Autodesk Inventor part; units mm, degrees
(part 2 of 3)
sketch "Sketch1" plane through (0, 0, 0) normal (0, 1, 0) x (-1, 0, 0)
  line L0 (1.875, 1.875) -> (-1.875, -1.875) construction
  circle A0 centre (0, 0) radius 5 projected
  circle A1 centre (0, 0) radius 7.7717
  line L1 (3.8714, 3.1643) -> (5.8376, 5.1305)
  line L2 (3.1643, 3.8714) -> (5.1305, 5.8376)
  line L3 (-3.1643, -3.8714) -> (-5.1305, -5.8376)
  line L4 (-3.8714, -3.1643) -> (-5.8376, -5.1305)
  line L5 (3.1643, -3.8714) -> (5.1305, -5.8376)
  line L6 (5.8376, -5.1305) -> (3.8714, -3.1643)
  line L7 (-3.8714, 3.1643) -> (-5.8376, 5.1305)
  line L8 (-3.1643, 3.8714) -> (-5.1305, 5.8376)
  line L9 (8.418, 2.4779) -> (8.489, 2.3785)
  line L10 (8.489, 2.3785) -> (8.5402, 2.3467)
  line L11 (8.5402, 2.3467) -> (8.588, 2.3267)
  line L12 (8.588, 2.3267) -> (8.6339, 2.3133)
  line L13 (8.6339, 2.3133) -> (8.6785, 2.3043)
  line L14 (8.6785, 2.3043) -> (8.7654, 2.2952)
  line L15 (8.7654, 2.2952) -> (8.8499, 2.2948)
  line L16 (8.8499, 2.2948) -> (8.9327, 2.3008)
  line L17 (8.9327, 2.3008) -> (9.0141, 2.3121)
  line L18 (9.0141, 2.3121) -> (9.1751, 2.3417)
  line L19 (9.1751, 2.3417) -> (9.3406, 2.3535)
  line L20 (9.3406, 2.3535) -> (9.5094, 2.3516)
  line L21 (9.5094, 2.3516) -> (9.6806, 2.3391)
  line L22 (9.6806, 2.3391) -> (9.8537, 2.3172)
  line L23 (9.8537, 2.3172) -> (10.0284, 2.2867)
  line L24 (10.0284, 2.2867) -> (10.2044, 2.2482)
  line L25 (10.2044, 2.2482) -> (10.3815, 2.202)
  line L26 (10.3815, 2.202) -> (10.5594, 2.1484)
  line L27 (10.5594, 2.1484) -> (10.7381, 2.0875)
  line L28 (10.7381, 2.0875) -> (10.9172, 2.0196)
  line L29 (10.9172, 2.0196) -> (11.0517, 1.9642)
  line L30 (11.0517, 1.9642) -> (11.1178, 1.5471)
  line L31 (11.1178, 1.5471) -> (11.007, 1.4528)
  line L32 (11.007, 1.4528) -> (10.8576, 1.3329)
  line L33 (10.8576, 1.3329) -> (10.7065, 1.2198)
  line L34 (10.7065, 1.2198) -> (10.5538, 1.1138)
  line L35 (10.5538, 1.1138) -> (10.3997, 1.0152)
  line L36 (10.3997, 1.0152) -> (10.2442, 0.9241)
  line L37 (10.2442, 0.9241) -> (10.0875, 0.8412)
  line L38 (10.0875, 0.8412) -> (9.9296, 0.7669)
  line L39 (9.9296, 0.7669) -> (9.7707, 0.702)
  line L40 (9.7707, 0.702) -> (9.6107, 0.6481)
  line L41 (9.6107, 0.6481) -> (9.4497, 0.6082)
  line L42 (9.4497, 0.6082) -> (9.2874, 0.5866)
  line L43 (9.2874, 0.5866) -> (9.2065, 0.5721)
  line L44 (9.2065, 0.5721) -> (9.1259, 0.5523)
  line L45 (9.1259, 0.5523) -> (9.0456, 0.5258)
  line L46 (9.0456, 0.5258) -> (8.9658, 0.4903)
  line L47 (8.9658, 0.4903) -> (8.9262, 0.4679)
  line L48 (8.9262, 0.4679) -> (8.8867, 0.441)
  line L49 (8.8867, 0.441) -> (8.8474, 0.4073)
  line L50 (8.8474, 0.4073) -> (8.8085, 0.3612)
  line L51 (8.8085, 0.3612) -> (8.7717, 0.2447)
  line L52 (8.7717, 0.2447) -> (8.7717, -0.2447)
  line L53 (8.7717, -0.2447) -> (8.8085, -0.3612)
  line L54 (8.8085, -0.3612) -> (8.8474, -0.4073)
  line L55 (8.8474, -0.4073) -> (8.8867, -0.441)
  line L56 (8.8867, -0.441) -> (8.9262, -0.4679)
  line L57 (8.9262, -0.4679) -> (8.9658, -0.4903)
  line L58 (8.9658, -0.4903) -> (9.0456, -0.5258)
  line L59 (9.0456, -0.5258) -> (9.1259, -0.5523)
  line L60 (9.1259, -0.5523) -> (9.2065, -0.5721)
  line L61 (9.2065, -0.5721) -> (9.2874, -0.5866)
  line L62 (9.2874, -0.5866) -> (9.4497, -0.6082)
  line L63 (9.4497, -0.6082) -> (9.6107, -0.6481)
  line L64 (9.6107, -0.6481) -> (9.7707, -0.702)
  line L65 (9.7707, -0.702) -> (9.9296, -0.7669)
  line L66 (9.9296, -0.7669) -> (10.0875, -0.8412)
  line L67 (10.0875, -0.8412) -> (10.2442, -0.9241)
  line L68 (10.2442, -0.9241) -> (10.3997, -1.0152)
  line L69 (10.3997, -1.0152) -> (10.5538, -1.1138)
  line L70 (10.5538, -1.1138) -> (10.7065, -1.2198)
  line L71 (10.7065, -1.2198) -> (10.8576, -1.3329)
  line L72 (10.8576, -1.3329) -> (11.007, -1.4528)
  line L73 (11.007, -1.4528) -> (11.1178, -1.5471)
  line L74 (11.1178, -1.5471) -> (11.0517, -1.9642)
  line L75 (11.0517, -1.9642) -> (10.9172, -2.0197)
  line L76 (10.9172, -2.0197) -> (10.7381, -2.0875)
  line L77 (10.7381, -2.0875) -> (10.5594, -2.1484)
  line L78 (10.5594, -2.1484) -> (10.3815, -2.202)
  line L79 (10.3815, -2.202) -> (10.2044, -2.2482)
  line L80 (10.2044, -2.2482) -> (10.0284, -2.2867)
  line L81 (10.0284, -2.2867) -> (9.8537, -2.3172)
  line L82 (9.8537, -2.3172) -> (9.6806, -2.3391)
  line L83 (9.6806, -2.3391) -> (9.5094, -2.3516)
  line L84 (9.5094, -2.3516) -> (9.3406, -2.3535)
  line L85 (9.3406, -2.3535) -> (9.1751, -2.3417)
  line L86 (9.1751, -2.3417) -> (9.0141, -2.3121)
  line L87 (9.0141, -2.3121) -> (8.9327, -2.3008)
  line L88 (8.9327, -2.3008) -> (8.8499, -2.2948)
  line L89 (8.8499, -2.2948) -> (8.7654, -2.2952)
  line L90 (8.7654, -2.2952) -> (8.6786, -2.3043)
  line L91 (8.6786, -2.3043) -> (8.6339, -2.3133)
  line L92 (8.6339, -2.3133) -> (8.588, -2.3268)
  line L93 (8.588, -2.3268) -> (8.5402, -2.3467)
  line L94 (8.5402, -2.3467) -> (8.489, -2.3785)
  line L95 (8.489, -2.3785) -> (8.418, -2.4779)
  line L96 (8.418, -2.4779) -> (8.2667, -2.9433)
  line L97 (8.2667, -2.9433) -> (8.2658, -3.0655)
  line L98 (8.2658, -3.0655) -> (8.2885, -3.1213)
  line L99 (8.2885, -3.1213) -> (8.3154, -3.1655)
  line L100 (8.3154, -3.1655) -> (8.3447, -3.2034)
  line L101 (8.3447, -3.2034) -> (8.3755, -3.2369)
  line L102 (8.3755, -3.2369) -> (8.4404, -3.2953)
  line L103 (8.4404, -3.2953) -> (8.5086, -3.3453)
  line L104 (8.5086, -3.3453) -> (8.5791, -3.3891)
  line L105 (8.5791, -3.3891) -> (8.6515, -3.4279)
  line L106 (8.6515, -3.4279) -> (8.7992, -3.4985)
  line L107 (8.7992, -3.4985) -> (8.94, -3.5863)
  line L108 (8.94, -3.5863) -> (9.0755, -3.687)
  line L109 (9.0755, -3.687) -> (9.2066, -3.7977)
  line L110 (9.2066, -3.7977) -> (9.3338, -3.9172)
  line L111 (9.3338, -3.9172) -> (9.4573, -4.0445)
  line L112 (9.4573, -4.0445) -> (9.577, -4.1792)
  line L113 (9.577, -4.1792) -> (9.6931, -4.3206)
  line L114 (9.6931, -4.3206) -> (9.8055, -4.4686)
  line L115 (9.8055, -4.4686) -> (9.9143, -4.6228)
  line L116 (9.9143, -4.6228) -> (10.0193, -4.783)
  line L117 (10.0193, -4.783) -> (10.0956, -4.907)
  line L118 (10.0956, -4.907) -> (9.9038, -5.2832)
  line L119 (9.9038, -5.2832) -> (9.7587, -5.2944)
  line L120 (9.7587, -5.2944) -> (9.5674, -5.3036)
  line L121 (9.5674, -5.3036) -> (9.3788, -5.3063)
  line L122 (9.3788, -5.3063) -> (9.1929, -5.3023)
  line L123 (9.1929, -5.3023) -> (9.0102, -5.2915)
  line L124 (9.0102, -5.2915) -> (8.8309, -5.2738)
  line L125 (8.8309, -5.2738) -> (8.6554, -5.2487)
  line L126 (8.6554, -5.2487) -> (8.484, -5.2161)
  line L127 (8.484, -5.2161) -> (8.3173, -5.1751)
  line L128 (8.3173, -5.1751) -> (8.1562, -5.1247)
  line L129 (8.1562, -5.1247) -> (8.0024, -5.0624)
  line L130 (8.0024, -5.0624) -> (7.8585, -4.9844)
  line L131 (7.8585, -4.9844) -> (7.7845, -4.9486)
  line L132 (7.7845, -4.9486) -> (7.7076, -4.9173)
  line L133 (7.7076, -4.9173) -> (7.6271, -4.8915)
  line L134 (7.6271, -4.8915) -> (7.5417, -4.8733)
  line L135 (7.5417, -4.8733) -> (7.4964, -4.8681)
  line L136 (7.4964, -4.8681) -> (7.4486, -4.8667)
  line L137 (7.4486, -4.8667) -> (7.3971, -4.8709)
  line L138 (7.3971, -4.8709) -> (7.3385, -4.8853)
  line L139 (7.3385, -4.8853) -> (7.2403, -4.9579)
  line L140 (7.2403, -4.9579) -> (6.9526, -5.3538)
  line L141 (6.9526, -5.3538) -> (6.914, -5.4697)
  line L142 (6.914, -5.4697) -> (6.9183, -5.5298)
  line L143 (6.9183, -5.5298) -> (6.9303, -5.5802)
  line L144 (6.9303, -5.5802) -> (6.9464, -5.6252)
  line L145 (6.9464, -5.6252) -> (6.9653, -5.6667)
  line L146 (6.9653, -5.6667) -> (7.009, -5.7423)
  line L147 (7.009, -5.7423) -> (7.0584, -5.8109)
  line L148 (7.0584, -5.8109) -> (7.1119, -5.8743)
  line L149 (7.1119, -5.8743) -> (7.1688, -5.9336)
  line L150 (7.1688, -5.9336) -> (7.2875, -6.0464)
  line L151 (7.2875, -6.0464) -> (7.3943, -6.1734)
  line L152 (7.3943, -6.1734) -> (7.492, -6.311)
  line L153 (7.492, -6.311) -> (7.5825, -6.4569)
  line L154 (7.5825, -6.4569) -> (7.6665, -6.6098)
  line L155 (7.6665, -6.6098) -> (7.7445, -6.769)
  line L156 (7.7445, -6.769) -> (7.8168, -6.9341)
  line L157 (7.8168, -6.9341) -> (7.8835, -7.1045)
  line L158 (7.8835, -7.1045) -> (7.9447, -7.28)
  line L159 (7.9447, -7.28) -> (8.0005, -7.4603)
  line L160 (8.0005, -7.4603) -> (8.0509, -7.6451)
  line L161 (8.0509, -7.6451) -> (8.0851, -7.7865)
  line L162 (8.0851, -7.7865) -> (7.7865, -8.0851)
  line L163 (7.7865, -8.0851) -> (7.6451, -8.0509)
  line L164 (7.6451, -8.0509) -> (7.4603, -8.0005)
  line L165 (7.4603, -8.0005) -> (7.28, -7.9447)
  line L166 (7.28, -7.9447) -> (7.1045, -7.8835)
  line L167 (7.1045, -7.8835) -> (6.9341, -7.8168)
  line L168 (6.9341, -7.8168) -> (6.769, -7.7445)
  line L169 (6.769, -7.7445) -> (6.6098, -7.6665)
  line L170 (6.6098, -7.6665) -> (6.4569, -7.5825)
  line L171 (6.4569, -7.5825) -> (6.311, -7.492)
  line L172 (6.311, -7.492) -> (6.1734, -7.3943)
  line L173 (6.1734, -7.3943) -> (6.0464, -7.2875)
  line L174 (6.0464, -7.2875) -> (5.9336, -7.1688)
  line L175 (5.9336, -7.1688) -> (5.8743, -7.1119)
  line L176 (5.8743, -7.1119) -> (5.8109, -7.0584)
  line L177 (5.8109, -7.0584) -> (5.7423, -7.009)
  line L178 (5.7423, -7.009) -> (5.6667, -6.9653)
  line L179 (5.6667, -6.9653) -> (5.6252, -6.9464)
  line L180 (5.6252, -6.9464) -> (5.5802, -6.9303)
  line L181 (5.5802, -6.9303) -> (5.5298, -6.9183)
  line L182 (5.5298, -6.9183) -> (5.4697, -6.9139)
  line L183 (5.4697, -6.9139) -> (5.3538, -6.9526)
  line L184 (5.3538, -6.9526) -> (4.9579, -7.2403)
  line L185 (4.9579, -7.2403) -> (4.8853, -7.3385)
  line L186 (4.8853, -7.3385) -> (4.8709, -7.3971)
  line L187 (4.8709, -7.3971) -> (4.8667, -7.4486)
  line L188 (4.8667, -7.4486) -> (4.8681, -7.4965)
  line L189 (4.8681, -7.4965) -> (4.8733, -7.5417)
  line L190 (4.8733, -7.5417) -> (4.8915, -7.6271)
  line L191 (4.8915, -7.6271) -> (4.9172, -7.7076)
  line L192 (4.9172, -7.7076) -> (4.9486, -7.7845)
  line L193 (4.9486, -7.7845) -> (4.9844, -7.8585)
  line L194 (4.9844, -7.8585) -> (5.0624, -8.0024)
  line L195 (5.0624, -8.0024) -> (5.1247, -8.1562)
  line L196 (5.1247, -8.1562) -> (5.1751, -8.3173)
  line L197 (5.1751, -8.3173) -> (5.2161, -8.484)
  line L198 (5.2161, -8.484) -> (5.2487, -8.6554)
  line L199 (5.2487, -8.6554) -> (5.2738, -8.8309)
  line L200 (5.2738, -8.8309) -> (5.2915, -9.0102)
  line L201 (5.2915, -9.0102) -> (5.3023, -9.1929)
  line L202 (5.3023, -9.1929) -> (5.3063, -9.3788)
  line L203 (5.3063, -9.3788) -> (5.3036, -9.5674)
  line L204 (5.3036, -9.5674) -> (5.2944, -9.7587)
  line L205 (5.2944, -9.7587) -> (5.2832, -9.9038)
  line L206 (5.2832, -9.9038) -> (4.907, -10.0956)
  line L207 (4.907, -10.0956) -> (4.783, -10.0193)
  line L208 (4.783, -10.0193) -> (4.6228, -9.9143)
  line L209 (4.6228, -9.9143) -> (4.4686, -9.8055)
  line L210 (4.4686, -9.8055) -> (4.3207, -9.6931)
  line L211 (4.3207, -9.6931) -> (4.1792, -9.577)
  line L212 (4.1792, -9.577) -> (4.0445, -9.4572)
  line L213 (4.0445, -9.4572) -> (3.9172, -9.3338)
  line L214 (3.9172, -9.3338) -> (3.7977, -9.2066)
  line L215 (3.7977, -9.2066) -> (3.687, -9.0755)
  line L216 (3.687, -9.0755) -> (3.5863, -8.94)
  line L217 (3.5863, -8.94) -> (3.4985, -8.7992)
  line L218 (3.4985, -8.7992) -> (3.4279, -8.6515)
  line L219 (3.4279, -8.6515) -> (3.3891, -8.5791)
  line L220 (3.3891, -8.5791) -> (3.3453, -8.5086)
  line L221 (3.3453, -8.5086) -> (3.2953, -8.4404)
  line L222 (3.2953, -8.4404) -> (3.2369, -8.3755)
  line L223 (3.2369, -8.3755) -> (3.2033, -8.3447)
  line L224 (3.2033, -8.3447) -> (3.1655, -8.3154)
  line L225 (3.1655, -8.3154) -> (3.1213, -8.2885)
  line L226 (3.1213, -8.2885) -> (3.0655, -8.2658)
  line L227 (3.0655, -8.2658) -> (2.9433, -8.2667)
  line L228 (2.9433, -8.2667) -> (2.4779, -8.418)
  line L229 (2.4779, -8.418) -> (2.3785, -8.489)
  line L230 (2.3785, -8.489) -> (2.3467, -8.5402)
  line L231 (2.3467, -8.5402) -> (2.3267, -8.588)
  line L232 (2.3267, -8.588) -> (2.3133, -8.6339)
  line L233 (2.3133, -8.6339) -> (2.3043, -8.6785)
  line L234 (2.3043, -8.6785) -> (2.2952, -8.7654)
  line L235 (2.2952, -8.7654) -> (2.2948, -8.8499)
  line L236 (2.2948, -8.8499) -> (2.3008, -8.9327)
  line L237 (2.3008, -8.9327) -> (2.3121, -9.0141)
  line L238 (2.3121, -9.0141) -> (2.3417, -9.1751)
  line L239 (2.3417, -9.1751) -> (2.3535, -9.3406)
  line L240 (2.3535, -9.3406) -> (2.3516, -9.5094)
  line L241 (2.3516, -9.5094) -> (2.3391, -9.6806)
  line L242 (2.3391, -9.6806) -> (2.3172, -9.8537)
  line L243 (2.3172, -9.8537) -> (2.2867, -10.0284)
  line L244 (2.2867, -10.0284) -> (2.2482, -10.2044)
  line L245 (2.2482, -10.2044) -> (2.202, -10.3815)
  line L246 (2.202, -10.3815) -> (2.1484, -10.5594)
  line L247 (2.1484, -10.5594) -> (2.0875, -10.7381)
  line L248 (2.0875, -10.7381) -> (2.0196, -10.9172)
  line L249 (2.0196, -10.9172) -> (1.9642, -11.0517)
  line L250 (1.9642, -11.0517) -> (1.5471, -11.1178)
  line L251 (1.5471, -11.1178) -> (1.4528, -11.007)
  line L252 (1.4528, -11.007) -> (1.3329, -10.8576)
  line L253 (1.3329, -10.8576) -> (1.2198, -10.7065)
  line L254 (1.2198, -10.7065) -> (1.1138, -10.5538)
  line L255 (1.1138, -10.5538) -> (1.0152, -10.3997)
  line L256 (1.0152, -10.3997) -> (0.9241, -10.2442)
  line L257 (0.9241, -10.2442) -> (0.8412, -10.0875)
  line L258 (0.8412, -10.0875) -> (0.7669, -9.9296)
  line L259 (0.7669, -9.9296) -> (0.702, -9.7707)
  line L260 (0.702, -9.7707) -> (0.6481, -9.6107)
  line L261 (0.6481, -9.6107) -> (0.6082, -9.4497)
  line L262 (0.6082, -9.4497) -> (0.5866, -9.2874)
  line L263 (0.5866, -9.2874) -> (0.5721, -9.2065)
  line L264 (0.5721, -9.2065) -> (0.5523, -9.1259)
  line L265 (0.5523, -9.1259) -> (0.5258, -9.0456)
  line L266 (0.5258, -9.0456) -> (0.4903, -8.9658)
  line L267 (0.4903, -8.9658) -> (0.4679, -8.9262)
  line L268 (0.4679, -8.9262) -> (0.441, -8.8867)
  line L269 (0.441, -8.8867) -> (0.4073, -8.8474)
  line L270 (0.4073, -8.8474) -> (0.3612, -8.8085)
  line L271 (0.3612, -8.8085) -> (0.2447, -8.7717)
  line L272 (0.2447, -8.7717) -> (-0.2447, -8.7717)
  line L273 (-0.2447, -8.7717) -> (-0.3612, -8.8085)
  line L274 (-0.3612, -8.8085) -> (-0.4073, -8.8474)
  line L275 (-0.4073, -8.8474) -> (-0.441, -8.8866)
  line L276 (-0.441, -8.8866) -> (-0.4679, -8.9262)
  line L277 (-0.4679, -8.9262) -> (-0.4903, -8.9658)
  line L278 (-0.4903, -8.9658) -> (-0.5258, -9.0456)
  line L279 (-0.5258, -9.0456) -> (-0.5523, -9.1259)
  line L280 (-0.5523, -9.1259) -> (-0.5721, -9.2065)
  line L281 (-0.5721, -9.2065) -> (-0.5866, -9.2874)
  line L282 (-0.5866, -9.2874) -> (-0.6082, -9.4497)
  line L283 (-0.6082, -9.4497) -> (-0.6481, -9.6107)
  line L284 (-0.6481, -9.6107) -> (-0.702, -9.7707)
  line L285 (-0.702, -9.7707) -> (-0.7669, -9.9296)
  line L286 (-0.7669, -9.9296) -> (-0.8412, -10.0875)
  line L287 (-0.8412, -10.0875) -> (-0.9241, -10.2442)
  line L288 (-0.9241, -10.2442) -> (-1.0152, -10.3997)
  line L289 (-1.0152, -10.3997) -> (-1.1138, -10.5538)
  line L290 (-1.1138, -10.5538) -> (-1.2198, -10.7065)
  line L291 (-1.2198, -10.7065) -> (-1.3329, -10.8576)
  line L292 (-1.3329, -10.8576) -> (-1.4528, -11.007)
  line L293 (-1.4528, -11.007) -> (-1.5471, -11.1178)
  line L294 (-1.5471, -11.1178) -> (-1.9642, -11.0517)
  line L295 (-1.9642, -11.0517) -> (-2.0197, -10.9172)
  line L296 (-2.0197, -10.9172) -> (-2.0875, -10.7381)
  line L297 (-2.0875, -10.7381) -> (-2.1484, -10.5594)
  line L298 (-2.1484, -10.5594) -> (-2.202, -10.3815)
  line L299 (-2.202, -10.3815) -> (-2.2482, -10.2044)
  line L300 (-2.2482, -10.2044) -> (-2.2867, -10.0284)
  line L301 (-2.2867, -10.0284) -> (-2.3172, -9.8537)
  line L302 (-2.3172, -9.8537) -> (-2.3391, -9.6806)
  line L303 (-2.3391, -9.6806) -> (-2.3516, -9.5094)
  line L304 (-2.3516, -9.5094) -> (-2.3535, -9.3406)
  line L305 (-2.3535, -9.3406) -> (-2.3417, -9.1751)
  line L306 (-2.3417, -9.1751) -> (-2.3121, -9.0141)
  line L307 (-2.3121, -9.0141) -> (-2.3008, -8.9327)
  line L308 (-2.3008, -8.9327) -> (-2.2948, -8.8499)
  line L309 (-2.2948, -8.8499) -> (-2.2952, -8.7654)
  line L310 (-2.2952, -8.7654) -> (-2.3043, -8.6785)
  line L311 (-2.3043, -8.6785) -> (-2.3133, -8.6339)
  line L312 (-2.3133, -8.6339) -> (-2.3267, -8.588)
  line L313 (-2.3267, -8.588) -> (-2.3467, -8.5402)
  line L314 (-2.3467, -8.5402) -> (-2.3785, -8.489)
  line L315 (-2.3785, -8.489) -> (-2.4779, -8.418)
  line L316 (-2.4779, -8.418) -> (-2.9433, -8.2667)
  line L317 (-2.9433, -8.2667) -> (-3.0655, -8.2658)
  line L318 (-3.0655, -8.2658) -> (-3.1213, -8.2885)
  line L319 (-3.1213, -8.2885) -> (-3.1655, -8.3154)
  line L320 (-3.1655, -8.3154) -> (-3.2033, -8.3447)
  line L321 (-3.2033, -8.3447) -> (-3.2369, -8.3755)
  line L322 (-3.2369, -8.3755) -> (-3.2953, -8.4404)
  line L323 (-3.2953, -8.4404) -> (-3.3453, -8.5086)
  line L324 (-3.3453, -8.5086) -> (-3.3891, -8.5791)
  line L325 (-3.3891, -8.5791) -> (-3.4279, -8.6515)
  line L326 (-3.4279, -8.6515) -> (-3.4985, -8.7992)
  line L327 (-3.4985, -8.7992) -> (-3.5863, -8.94)
  line L328 (-3.5863, -8.94) -> (-3.687, -9.0755)
  line L329 (-3.687, -9.0755) -> (-3.7977, -9.2066)
  line L330 (-3.7977, -9.2066) -> (-3.9172, -9.3338)
  line L331 (-3.9172, -9.3338) -> (-4.0445, -9.4572)
  line L332 (-4.0445, -9.4572) -> (-4.1792, -9.577)
  line L333 (-4.1792, -9.577) -> (-4.3206, -9.6931)
  line L334 (-4.3206, -9.6931) -> (-4.4686, -9.8055)
  line L335 (-4.4686, -9.8055) -> (-4.6228, -9.9143)
  line L336 (-4.6228, -9.9143) -> (-4.783, -10.0193)
  line L337 (-4.783, -10.0193) -> (-4.907, -10.0956)
  line L338 (-4.907, -10.0956) -> (-5.2832, -9.9038)
  line L339 (-5.2832, -9.9038) -> (-5.2944, -9.7587)
  line L340 (-5.2944, -9.7587) -> (-5.3036, -9.5674)
  line L341 (-5.3036, -9.5674) -> (-5.3063, -9.3788)
  line L342 (-5.3063, -9.3788) -> (-5.3023, -9.1929)
  line L343 (-5.3023, -9.1929) -> (-5.2915, -9.0102)
  line L344 (-5.2915, -9.0102) -> (-5.2738, -8.8309)
  line L345 (-5.2738, -8.8309) -> (-5.2487, -8.6554)
  line L346 (-5.2487, -8.6554) -> (-5.2161, -8.484)
  line L347 (-5.2161, -8.484) -> (-5.1751, -8.3173)
  line L348 (-5.1751, -8.3173) -> (-5.1247, -8.1562)
  line L349 (-5.1247, -8.1562) -> (-5.0624, -8.0024)
  line L350 (-5.0624, -8.0024) -> (-4.9844, -7.8584)
  line L351 (-4.9844, -7.8584) -> (-4.9486, -7.7845)
  line L352 (-4.9486, -7.7845) -> (-4.9173, -7.7076)
  line L353 (-4.9173, -7.7076) -> (-4.8915, -7.6271)
  line L354 (-4.8915, -7.6271) -> (-4.8733, -7.5417)
  line L355 (-4.8733, -7.5417) -> (-4.8681, -7.4965)
  line L356 (-4.8681, -7.4965) -> (-4.8667, -7.4486)
  line L357 (-4.8667, -7.4486) -> (-4.8709, -7.3971)
  line L358 (-4.8709, -7.3971) -> (-4.8853, -7.3385)
  line L359 (-4.8853, -7.3385) -> (-4.9579, -7.2403)
  line L360 (-4.9579, -7.2403) -> (-5.3538, -6.9526)
  line L361 (-5.3538, -6.9526) -> (-5.4697, -6.914)
  line L362 (-5.4697, -6.914) -> (-5.5298, -6.9183)
  line L363 (-5.5298, -6.9183) -> (-5.5802, -6.9303)
  line L364 (-5.5802, -6.9303) -> (-5.6252, -6.9464)
  line L365 (-5.6252, -6.9464) -> (-5.6667, -6.9653)
  line L366 (-5.6667, -6.9653) -> (-5.7423, -7.009)
  line L367 (-5.7423, -7.009) -> (-5.8109, -7.0584)
  line L368 (-5.8109, -7.0584) -> (-5.8743, -7.1119)
  line L369 (-5.8743, -7.1119) -> (-5.9336, -7.1688)
  line L370 (-5.9336, -7.1688) -> (-6.0464, -7.2875)
  line L371 (-6.0464, -7.2875) -> (-6.1734, -7.3943)
  line L372 (-6.1734, -7.3943) -> (-6.311, -7.492)
  line L373 (-6.311, -7.492) -> (-6.4569, -7.5825)
  line L374 (-6.4569, -7.5825) -> (-6.6098, -7.6665)
  line L375 (-6.6098, -7.6665) -> (-6.769, -7.7445)
  line L376 (-6.769, -7.7445) -> (-6.9341, -7.8168)
  line L377 (-6.9341, -7.8168) -> (-7.1045, -7.8835)
  line L378 (-7.1045, -7.8835) -> (-7.28, -7.9447)
  line L379 (-7.28, -7.9447) -> (-7.4603, -8.0005)
  line L380 (-7.4603, -8.0005) -> (-7.6451, -8.0509)
  line L381 (-7.6451, -8.0509) -> (-7.7865, -8.0851)
  line L382 (-7.7865, -8.0851) -> (-8.0851, -7.7865)
  line L383 (-8.0851, -7.7865) -> (-8.0509, -7.6451)
  line L384 (-8.0509, -7.6451) -> (-8.0005, -7.4603)
  line L385 (-8.0005, -7.4603) -> (-7.9447, -7.28)
  line L386 (-7.9447, -7.28) -> (-7.8835, -7.1045)
  line L387 (-7.8835, -7.1045) -> (-7.8168, -6.9341)
  line L388 (-7.8168, -6.9341) -> (-7.7445, -6.769)
  line L389 (-7.7445, -6.769) -> (-7.6665, -6.6098)
  line L390 (-7.6665, -6.6098) -> (-7.5825, -6.4569)
  line L391 (-7.5825, -6.4569) -> (-7.492, -6.311)
  line L392 (-7.492, -6.311) -> (-7.3943, -6.1734)
  line L393 (-7.3943, -6.1734) -> (-7.2875, -6.0464)
  line L394 (-7.2875, -6.0464) -> (-7.1688, -5.9336)
  line L395 (-7.1688, -5.9336) -> (-7.1119, -5.8743)
  line L396 (-7.1119, -5.8743) -> (-7.0584, -5.8108)
  line L397 (-7.0584, -5.8108) -> (-7.009, -5.7423)
  line L398 (-7.009, -5.7423) -> (-6.9653, -5.6667)
  line L399 (-6.9653, -5.6667) -> (-6.9464, -5.6252)
  line L400 (-6.9464, -5.6252) -> (-6.9303, -5.5802)
  line L401 (-6.9303, -5.5802) -> (-6.9183, -5.5298)
  line L402 (-6.9183, -5.5298) -> (-6.9139, -5.4697)
  line L403 (-6.9139, -5.4697) -> (-6.9526, -5.3538)
  line L404 (-6.9526, -5.3538) -> (-7.2403, -4.9579)
  line L405 (-7.2403, -4.9579) -> (-7.3385, -4.8853)
  line L406 (-7.3385, -4.8853) -> (-7.3971, -4.8709)
  line L407 (-7.3971, -4.8709) -> (-7.4486, -4.8667)
  line L408 (-7.4486, -4.8667) -> (-7.4965, -4.8681)
  line L409 (-7.4965, -4.8681) -> (-7.5417, -4.8733)
  line L410 (-7.5417, -4.8733) -> (-7.6271, -4.8915)
  line L411 (-7.6271, -4.8915) -> (-7.7076, -4.9173)
  line L412 (-7.7076, -4.9173) -> (-7.7845, -4.9486)
  line L413 (-7.7845, -4.9486) -> (-7.8585, -4.9844)
  line L414 (-7.8585, -4.9844) -> (-8.0024, -5.0624)
  line L415 (-8.0024, -5.0624) -> (-8.1562, -5.1247)
  line L416 (-8.1562, -5.1247) -> (-8.3173, -5.1751)
  line L417 (-8.3173, -5.1751) -> (-8.484, -5.2161)
  line L418 (-8.484, -5.2161) -> (-8.6554, -5.2487)
  line L419 (-8.6554, -5.2487) -> (-8.8309, -5.2737)
  line L420 (-8.8309, -5.2737) -> (-9.0102, -5.2915)
  line L421 (-9.0102, -5.2915) -> (-9.1929, -5.3023)
  line L422 (-9.1929, -5.3023) -> (-9.3788, -5.3063)
  line L423 (-9.3788, -5.3063) -> (-9.5674, -5.3036)
  line L424 (-9.5674, -5.3036) -> (-9.7587, -5.2944)
  line L425 (-9.7587, -5.2944) -> (-9.9038, -5.2832)
  line L426 (-9.9038, -5.2832) -> (-10.0956, -4.907)
  line L427 (-10.0956, -4.907) -> (-10.0193, -4.783)
  line L428 (-10.0193, -4.783) -> (-9.9143, -4.6228)
  line L429 (-9.9143, -4.6228) -> (-9.8055, -4.4686)
  line L430 (-9.8055, -4.4686) -> (-9.6931, -4.3206)
  line L431 (-9.6931, -4.3206) -> (-9.577, -4.1792)
  line L432 (-9.577, -4.1792) -> (-9.4572, -4.0445)
  line L433 (-9.4572, -4.0445) -> (-9.3338, -3.9172)
  line L434 (-9.3338, -3.9172) -> (-9.2066, -3.7977)
  line L435 (-9.2066, -3.7977) -> (-9.0755, -3.687)
  line L436 (-9.0755, -3.687) -> (-8.94, -3.5863)
  line L437 (-8.94, -3.5863) -> (-8.7992, -3.4985)
  line L438 (-8.7992, -3.4985) -> (-8.6515, -3.4279)
  line L439 (-8.6515, -3.4279) -> (-8.5791, -3.3891)
  line L440 (-8.5791, -3.3891) -> (-8.5086, -3.3453)
  line L441 (-8.5086, -3.3453) -> (-8.4404, -3.2953)
  line L442 (-8.4404, -3.2953) -> (-8.3755, -3.2369)
  line L443 (-8.3755, -3.2369) -> (-8.3447, -3.2034)
  line L444 (-8.3447, -3.2034) -> (-8.3154, -3.1655)
  line L445 (-8.3154, -3.1655) -> (-8.2885, -3.1213)
  line L446 (-8.2885, -3.1213) -> (-8.2658, -3.0655)
  line L447 (-8.2658, -3.0655) -> (-8.2667, -2.9433)
  line L448 (-8.2667, -2.9433) -> (-8.418, -2.4779)
  line L449 (-8.418, -2.4779) -> (-8.489, -2.3785)
  line L450 (-8.489, -2.3785) -> (-8.5402, -2.3467)
  line L451 (-8.5402, -2.3467) -> (-8.588, -2.3267)
  line L452 (-8.588, -2.3267) -> (-8.6339, -2.3133)
  line L453 (-8.6339, -2.3133) -> (-8.6786, -2.3043)
  line L454 (-8.6786, -2.3043) -> (-8.7654, -2.2952)
  line L455 (-8.7654, -2.2952) -> (-8.8499, -2.2948)
  line L456 (-8.8499, -2.2948) -> (-8.9327, -2.3009)
  line L457 (-8.9327, -2.3009) -> (-9.0141, -2.3121)
  line L458 (-9.0141, -2.3121) -> (-9.1751, -2.3417)
  line L459 (-9.1751, -2.3417) -> (-9.3406, -2.3535)
  line L460 (-9.3406, -2.3535) -> (-9.5094, -2.3516)
  line L461 (-9.5094, -2.3516) -> (-9.6806, -2.3391)
  line L462 (-9.6806, -2.3391) -> (-9.8537, -2.3172)
  line L463 (-9.8537, -2.3172) -> (-10.0284, -2.2867)
  line L464 (-10.0284, -2.2867) -> (-10.2044, -2.2482)
  line L465 (-10.2044, -2.2482) -> (-10.3815, -2.202)
  line L466 (-10.3815, -2.202) -> (-10.5594, -2.1484)
  line L467 (-10.5594, -2.1484) -> (-10.7381, -2.0875)
  line L468 (-10.7381, -2.0875) -> (-10.9172, -2.0197)
  line L469 (-10.9172, -2.0197) -> (-11.0517, -1.9642)
  line L470 (-11.0517, -1.9642) -> (-11.1178, -1.5471)
  line L471 (-11.1178, -1.5471) -> (-11.007, -1.4528)
  line L472 (-11.007, -1.4528) -> (-10.8576, -1.3329)
  line L473 (-10.8576, -1.3329) -> (-10.7065, -1.2198)
  line L474 (-10.7065, -1.2198) -> (-10.5538, -1.1138)
  line L475 (-10.5538, -1.1138) -> (-10.3997, -1.0152)
  line L476 (-10.3997, -1.0152) -> (-10.2442, -0.9241)
  line L477 (-10.2442, -0.9241) -> (-10.0875, -0.8412)
  line L478 (-10.0875, -0.8412) -> (-9.9296, -0.7669)
  line L479 (-9.9296, -0.7669) -> (-9.7707, -0.702)
  line L480 (-9.7707, -0.702) -> (-9.6107, -0.6481)
  line L481 (-9.6107, -0.6481) -> (-9.4497, -0.6082)
  line L482 (-9.4497, -0.6082) -> (-9.2874, -0.5866)
  line L483 (-9.2874, -0.5866) -> (-9.2065, -0.5721)
  line L484 (-9.2065, -0.5721) -> (-9.1259, -0.5523)
  line L485 (-9.1259, -0.5523) -> (-9.0456, -0.5258)
  line L486 (-9.0456, -0.5258) -> (-8.9658, -0.4903)
  line L487 (-8.9658, -0.4903) -> (-8.9262, -0.4679)
  line L488 (-8.9262, -0.4679) -> (-8.8867, -0.441)
  line L489 (-8.8867, -0.441) -> (-8.8474, -0.4073)
  line L490 (-8.8474, -0.4073) -> (-8.8085, -0.3612)
  line L491 (-8.8085, -0.3612) -> (-8.7717, -0.2447)
  line L492 (-8.7717, -0.2447) -> (-8.7717, 0.2447)
  line L493 (-8.7717, 0.2447) -> (-8.8085, 0.3612)
  line L494 (-8.8085, 0.3612) -> (-8.8474, 0.4073)
  line L495 (-8.8474, 0.4073) -> (-8.8866, 0.441)
  line L496 (-8.8866, 0.441) -> (-8.9262, 0.4679)
  line L497 (-8.9262, 0.4679) -> (-8.9658, 0.4903)
  line L498 (-8.9658, 0.4903) -> (-9.0456, 0.5258)
  line L499 (-9.0456, 0.5258) -> (-9.1259, 0.5523)
  line L500 (-9.1259, 0.5523) -> (-9.2065, 0.5721)
  line L501 (-9.2065, 0.5721) -> (-9.2874, 0.5866)
  line L502 (-9.2874, 0.5866) -> (-9.4497, 0.6082)
  line L503 (-9.4497, 0.6082) -> (-9.6107, 0.6481)
  line L504 (-9.6107, 0.6481) -> (-9.7707, 0.702)
  line L505 (-9.7707, 0.702) -> (-9.9296, 0.7669)
  line L506 (-9.9296, 0.7669) -> (-10.0875, 0.8412)
  line L507 (-10.0875, 0.8412) -> (-10.2442, 0.9241)
  line L508 (-10.2442, 0.9241) -> (-10.3997, 1.0152)
  line L509 (-10.3997, 1.0152) -> (-10.5538, 1.1139)
  line L510 (-10.5538, 1.1139) -> (-10.7065, 1.2198)
  line L511 (-10.7065, 1.2198) -> (-10.8576, 1.3329)
  line L512 (-10.8576, 1.3329) -> (-11.007, 1.4528)
  line L513 (-11.007, 1.4528) -> (-11.1178, 1.5471)
  line L514 (-11.1178, 1.5471) -> (-11.0517, 1.9642)
  line L515 (-11.0517, 1.9642) -> (-10.9172, 2.0196)
  line L516 (-10.9172, 2.0196) -> (-10.7381, 2.0875)
  line L517 (-10.7381, 2.0875) -> (-10.5594, 2.1484)
  line L518 (-10.5594, 2.1484) -> (-10.3815, 2.202)
  line L519 (-10.3815, 2.202) -> (-10.2044, 2.2482)
  line L520 (-10.2044, 2.2482) -> (-10.0284, 2.2867)
  line L521 (-10.0284, 2.2867) -> (-9.8537, 2.3172)
  line L522 (-9.8537, 2.3172) -> (-9.6806, 2.3391)
  line L523 (-9.6806, 2.3391) -> (-9.5094, 2.3516)
  line L524 (-9.5094, 2.3516) -> (-9.3406, 2.3535)
  line L525 (-9.3406, 2.3535) -> (-9.1751, 2.3417)
  line L526 (-9.1751, 2.3417) -> (-9.0141, 2.3121)
  line L527 (-9.0141, 2.3121) -> (-8.9327, 2.3008)
  line L528 (-8.9327, 2.3008) -> (-8.8499, 2.2948)
  line L529 (-8.8499, 2.2948) -> (-8.7654, 2.2952)
  line L530 (-8.7654, 2.2952) -> (-8.6785, 2.3043)
  line L531 (-8.6785, 2.3043) -> (-8.6339, 2.3133)
  line L532 (-8.6339, 2.3133) -> (-8.588, 2.3267)
  line L533 (-8.588, 2.3267) -> (-8.5402, 2.3467)
  line L534 (-8.5402, 2.3467) -> (-8.489, 2.3785)
  line L535 (-8.489, 2.3785) -> (-8.418, 2.4779)
  line L536 (-8.418, 2.4779) -> (-8.2667, 2.9433)
  line L537 (-8.2667, 2.9433) -> (-8.2658, 3.0655)
  line L538 (-8.2658, 3.0655) -> (-8.2885, 3.1213)
  line L539 (-8.2885, 3.1213) -> (-8.3154, 3.1655)
  line L540 (-8.3154, 3.1655) -> (-8.3447, 3.2033)
  line L541 (-8.3447, 3.2033) -> (-8.3755, 3.2369)
  line L542 (-8.3755, 3.2369) -> (-8.4404, 3.2953)
  line L543 (-8.4404, 3.2953) -> (-8.5086, 3.3453)
  line L544 (-8.5086, 3.3453) -> (-8.5791, 3.3891)
  line L545 (-8.5791, 3.3891) -> (-8.6515, 3.4279)
  line L546 (-8.6515, 3.4279) -> (-8.7992, 3.4985)
  line L547 (-8.7992, 3.4985) -> (-8.94, 3.5863)
  line L548 (-8.94, 3.5863) -> (-9.0755, 3.687)
  line L549 (-9.0755, 3.687) -> (-9.2066, 3.7977)
  line L550 (-9.2066, 3.7977) -> (-9.3338, 3.9172)
  line L551 (-9.3338, 3.9172) -> (-9.4572, 4.0445)
  line L552 (-9.4572, 4.0445) -> (-9.577, 4.1792)
  line L553 (-9.577, 4.1792) -> (-9.6931, 4.3207)
  line L554 (-9.6931, 4.3207) -> (-9.8055, 4.4686)
  line L555 (-9.8055, 4.4686) -> (-9.9143, 4.6228)
  line L556 (-9.9143, 4.6228) -> (-10.0193, 4.783)
  line L557 (-10.0193, 4.783) -> (-10.0956, 4.907)
  line L558 (-10.0956, 4.907) -> (-9.9038, 5.2832)
  line L559 (-9.9038, 5.2832) -> (-9.7587, 5.2944)
  line L560 (-9.7587, 5.2944) -> (-9.5674, 5.3036)
  line L561 (-9.5674, 5.3036) -> (-9.3788, 5.3063)
  line L562 (-9.3788, 5.3063) -> (-9.1929, 5.3023)
  line L563 (-9.1929, 5.3023) -> (-9.0102, 5.2915)
  line L564 (-9.0102, 5.2915) -> (-8.8309, 5.2737)
  line L565 (-8.8309, 5.2737) -> (-8.6554, 5.2487)
  line L566 (-8.6554, 5.2487) -> (-8.484, 5.2161)
  line L567 (-8.484, 5.2161) -> (-8.3173, 5.1751)
  line L568 (-8.3173, 5.1751) -> (-8.1562, 5.1247)
  line L569 (-8.1562, 5.1247) -> (-8.0024, 5.0624)
  line L570 (-8.0024, 5.0624) -> (-7.8585, 4.9844)
  line L571 (-7.8585, 4.9844) -> (-7.7845, 4.9486)
  line L572 (-7.7845, 4.9486) -> (-7.7076, 4.9172)
  line L573 (-7.7076, 4.9172) -> (-7.6271, 4.8915)
  line L574 (-7.6271, 4.8915) -> (-7.5417, 4.8733)
  line L575 (-7.5417, 4.8733) -> (-7.4965, 4.8681)
  line L576 (-7.4965, 4.8681) -> (-7.4486, 4.8667)
  line L577 (-7.4486, 4.8667) -> (-7.3971, 4.8709)
  line L578 (-7.3971, 4.8709) -> (-7.3385, 4.8853)
  line L579 (-7.3385, 4.8853) -> (-7.2403, 4.9579)
  line L580 (-7.2403, 4.9579) -> (-6.9526, 5.3538)
  line L581 (-6.9526, 5.3538) -> (-6.914, 5.4697)
  line L582 (-6.914, 5.4697) -> (-6.9183, 5.5298)
  line L583 (-6.9183, 5.5298) -> (-6.9303, 5.5802)
  line L584 (-6.9303, 5.5802) -> (-6.9464, 5.6252)
  line L585 (-6.9464, 5.6252) -> (-6.9653, 5.6667)
  line L586 (-6.9653, 5.6667) -> (-7.009, 5.7423)
  line L587 (-7.009, 5.7423) -> (-7.0584, 5.8109)
  line L588 (-7.0584, 5.8109) -> (-7.1119, 5.8743)
  line L589 (-7.1119, 5.8743) -> (-7.1688, 5.9336)
  line L590 (-7.1688, 5.9336) -> (-7.2875, 6.0464)
  line L591 (-7.2875, 6.0464) -> (-7.3943, 6.1734)
  line L592 (-7.3943, 6.1734) -> (-7.492, 6.311)
  line L593 (-7.492, 6.311) -> (-7.5825, 6.4569)
  line L594 (-7.5825, 6.4569) -> (-7.6665, 6.6098)
  line L595 (-7.6665, 6.6098) -> (-7.7445, 6.769)
  line L596 (-7.7445, 6.769) -> (-7.8168, 6.9341)
  line L597 (-7.8168, 6.9341) -> (-7.8835, 7.1045)
  line L598 (-7.8835, 7.1045) -> (-7.9447, 7.28)
  line L599 (-7.9447, 7.28) -> (-8.0005, 7.4603)
  line L600 (-8.0005, 7.4603) -> (-8.0509, 7.6451)
  line L601 (-8.0509, 7.6451) -> (-8.0851, 7.7865)
  line L602 (-8.0851, 7.7865) -> (-7.7865, 8.0851)
  line L603 (-7.7865, 8.0851) -> (-7.6451, 8.0509)
  line L604 (-7.6451, 8.0509) -> (-7.4603, 8.0005)
  line L605 (-7.4603, 8.0005) -> (-7.28, 7.9447)
  line L606 (-7.28, 7.9447) -> (-7.1045, 7.8835)
  line L607 (-7.1045, 7.8835) -> (-6.9341, 7.8168)
  line L608 (-6.9341, 7.8168) -> (-6.769, 7.7446)
  line L609 (-6.769, 7.7446) -> (-6.6098, 7.6665)
  line L610 (-6.6098, 7.6665) -> (-6.4569, 7.5825)
  line L611 (-6.4569, 7.5825) -> (-6.311, 7.492)
  line L612 (-6.311, 7.492) -> (-6.1734, 7.3942)
  line L613 (-6.1734, 7.3942) -> (-6.0464, 7.2875)
  line L614 (-6.0464, 7.2875) -> (-5.9336, 7.1688)
  line L615 (-5.9336, 7.1688) -> (-5.8743, 7.1119)
  line L616 (-5.8743, 7.1119) -> (-5.8108, 7.0584)
  line L617 (-5.8108, 7.0584) -> (-5.7423, 7.009)
  line L618 (-5.7423, 7.009) -> (-5.6667, 6.9653)
  line L619 (-5.6667, 6.9653) -> (-5.6252, 6.9464)
  line L620 (-5.6252, 6.9464) -> (-5.5802, 6.9303)
  line L621 (-5.5802, 6.9303) -> (-5.5298, 6.9183)
  line L622 (-5.5298, 6.9183) -> (-5.4697, 6.914)
  line L623 (-5.4697, 6.914) -> (-5.3538, 6.9526)
  line L624 (-5.3538, 6.9526) -> (-4.9579, 7.2403)
  line L625 (-4.9579, 7.2403) -> (-4.8853, 7.3385)
  line L626 (-4.8853, 7.3385) -> (-4.8709, 7.3971)
  line L627 (-4.8709, 7.3971) -> (-4.8667, 7.4486)
  line L628 (-4.8667, 7.4486) -> (-4.8681, 7.4964)
  line L629 (-4.8681, 7.4964) -> (-4.8733, 7.5417)
  line L630 (-4.8733, 7.5417) -> (-4.8915, 7.6271)
  line L631 (-4.8915, 7.6271) -> (-4.9173, 7.7076)
  line L632 (-4.9173, 7.7076) -> (-4.9486, 7.7845)
  line L633 (-4.9486, 7.7845) -> (-4.9844, 7.8585)
  line L634 (-4.9844, 7.8585) -> (-5.0624, 8.0024)
  line L635 (-5.0624, 8.0024) -> (-5.1247, 8.1562)
  line L636 (-5.1247, 8.1562) -> (-5.1751, 8.3173)
  line L637 (-5.1751, 8.3173) -> (-5.2161, 8.484)
  line L638 (-5.2161, 8.484) -> (-5.2487, 8.6554)
  line L639 (-5.2487, 8.6554) -> (-5.2737, 8.8309)
  line L640 (-5.2737, 8.8309) -> (-5.2915, 9.0102)
  line L641 (-5.2915, 9.0102) -> (-5.3023, 9.1929)
  line L642 (-5.3023, 9.1929) -> (-5.3063, 9.3787)
  line L643 (-5.3063, 9.3787) -> (-5.3036, 9.5674)
  line L644 (-5.3036, 9.5674) -> (-5.2944, 9.7587)
  line L645 (-5.2944, 9.7587) -> (-5.2832, 9.9038)
  line L646 (-5.2832, 9.9038) -> (-4.907, 10.0956)
  line L647 (-4.907, 10.0956) -> (-4.783, 10.0193)
  line L648 (-4.783, 10.0193) -> (-4.6228, 9.9143)
  line L649 (-4.6228, 9.9143) -> (-4.4686, 9.8055)
  line L650 (-4.4686, 9.8055) -> (-4.3206, 9.6931)
  line L651 (-4.3206, 9.6931) -> (-4.1792, 9.577)
  line L652 (-4.1792, 9.577) -> (-4.0445, 9.4573)
  line L653 (-4.0445, 9.4573) -> (-3.9172, 9.3338)
  line L654 (-3.9172, 9.3338) -> (-3.7977, 9.2066)
  line L655 (-3.7977, 9.2066) -> (-3.687, 9.0755)
  line L656 (-3.687, 9.0755) -> (-3.5863, 8.94)
  line L657 (-3.5863, 8.94) -> (-3.4985, 8.7992)
  line L658 (-3.4985, 8.7992) -> (-3.4279, 8.6516)
  line L659 (-3.4279, 8.6516) -> (-3.3891, 8.5791)
  line L660 (-3.3891, 8.5791) -> (-3.3453, 8.5086)
  line L661 (-3.3453, 8.5086) -> (-3.2953, 8.4404)
  line L662 (-3.2953, 8.4404) -> (-3.2369, 8.3755)
  line L663 (-3.2369, 8.3755) -> (-3.2034, 8.3447)
  line L664 (-3.2034, 8.3447) -> (-3.1655, 8.3154)
  line L665 (-3.1655, 8.3154) -> (-3.1213, 8.2885)
  line L666 (-3.1213, 8.2885) -> (-3.0655, 8.2658)
  line L667 (-3.0655, 8.2658) -> (-2.9433, 8.2667)
  line L668 (-2.9433, 8.2667) -> (-2.4779, 8.418)
  line L669 (-2.4779, 8.418) -> (-2.3785, 8.489)
  line L670 (-2.3785, 8.489) -> (-2.3467, 8.5402)
  line L671 (-2.3467, 8.5402) -> (-2.3267, 8.588)
  line L672 (-2.3267, 8.588) -> (-2.3133, 8.6339)
  line L673 (-2.3133, 8.6339) -> (-2.3042, 8.6785)
  line L674 (-2.3042, 8.6785) -> (-2.2952, 8.7654)
  line L675 (-2.2952, 8.7654) -> (-2.2948, 8.8499)
  line L676 (-2.2948, 8.8499) -> (-2.3008, 8.9327)
  line L677 (-2.3008, 8.9327) -> (-2.3121, 9.0141)
  line L678 (-2.3121, 9.0141) -> (-2.3417, 9.1751)
  line L679 (-2.3417, 9.1751) -> (-2.3535, 9.3406)
  line L680 (-2.3535, 9.3406) -> (-2.3516, 9.5094)
  line L681 (-2.3516, 9.5094) -> (-2.3391, 9.6806)
  line L682 (-2.3391, 9.6806) -> (-2.3172, 9.8537)
  line L683 (-2.3172, 9.8537) -> (-2.2867, 10.0284)
  line L684 (-2.2867, 10.0284) -> (-2.2482, 10.2044)
  line L685 (-2.2482, 10.2044) -> (-2.202, 10.3815)
  line L686 (-2.202, 10.3815) -> (-2.1484, 10.5594)
  line L687 (-2.1484, 10.5594) -> (-2.0875, 10.7381)
  line L688 (-2.0875, 10.7381) -> (-2.0197, 10.9172)
  line L689 (-2.0197, 10.9172) -> (-1.9642, 11.0517)
  line L690 (-1.9642, 11.0517) -> (-1.5471, 11.1178)
  line L691 (-1.5471, 11.1178) -> (-1.4528, 11.0069)
  line L692 (-1.4528, 11.0069) -> (-1.3329, 10.8576)
  line L693 (-1.3329, 10.8576) -> (-1.2198, 10.7065)
  line L694 (-1.2198, 10.7065) -> (-1.1138, 10.5538)
  line L695 (-1.1138, 10.5538) -> (-1.0152, 10.3997)
  line L696 (-1.0152, 10.3997) -> (-0.9241, 10.2442)
  line L697 (-0.9241, 10.2442) -> (-0.8412, 10.0875)
  line L698 (-0.8412, 10.0875) -> (-0.7669, 9.9296)
  line L699 (-0.7669, 9.9296) -> (-0.702, 9.7707)
  line L700 (-0.702, 9.7707) -> (-0.6481, 9.6107)
  line L701 (-0.6481, 9.6107) -> (-0.6082, 9.4497)
  line L702 (-0.6082, 9.4497) -> (-0.5866, 9.2874)
  line L703 (-0.5866, 9.2874) -> (-0.5721, 9.2065)
  line L704 (-0.5721, 9.2065) -> (-0.5523, 9.1259)
  line L705 (-0.5523, 9.1259) -> (-0.5258, 9.0456)
  line L706 (-0.5258, 9.0456) -> (-0.4903, 8.9658)
  line L707 (-0.4903, 8.9658) -> (-0.4679, 8.9262)
  line L708 (-0.4679, 8.9262) -> (-0.441, 8.8866)
  line L709 (-0.441, 8.8866) -> (-0.4073, 8.8474)
  line L710 (-0.4073, 8.8474) -> (-0.3612, 8.8085)
  line L711 (-0.3612, 8.8085) -> (-0.2447, 8.7717)
  line L712 (-0.2447, 8.7717) -> (0.2447, 8.7717)
  line L713 (0.2447, 8.7717) -> (0.3612, 8.8085)
  line L714 (0.3612, 8.8085) -> (0.4073, 8.8474)
  line L715 (0.4073, 8.8474) -> (0.441, 8.8867)
  line L716 (0.441, 8.8867) -> (0.4679, 8.9262)
  line L717 (0.4679, 8.9262) -> (0.4903, 8.9658)
  line L718 (0.4903, 8.9658) -> (0.5258, 9.0456)
  line L719 (0.5258, 9.0456) -> (0.5523, 9.1259)
  line L720 (0.5523, 9.1259) -> (0.5721, 9.2065)
  line L721 (0.5721, 9.2065) -> (0.5866, 9.2874)
  line L722 (0.5866, 9.2874) -> (0.6082, 9.4497)
  line L723 (0.6082, 9.4497) -> (0.6481, 9.6107)
  line L724 (0.6481, 9.6107) -> (0.702, 9.7707)
  line L725 (0.702, 9.7707) -> (0.7669, 9.9296)
  line L726 (0.7669, 9.9296) -> (0.8412, 10.0875)
  line L727 (0.8412, 10.0875) -> (0.9241, 10.2442)
  line L728 (0.9241, 10.2442) -> (1.0152, 10.3997)
  line L729 (1.0152, 10.3997) -> (1.1139, 10.5538)
  line L730 (1.1139, 10.5538) -> (1.2198, 10.7065)
  line L731 (1.2198, 10.7065) -> (1.3329, 10.8576)
  line L732 (1.3329, 10.8576) -> (1.4528, 11.007)
  line L733 (1.4528, 11.007) -> (1.5471, 11.1178)
  line L734 (1.5471, 11.1178) -> (1.9642, 11.0517)
  line L735 (1.9642, 11.0517) -> (2.0196, 10.9172)
  line L736 (2.0196, 10.9172) -> (2.0875, 10.7381)
  line L737 (2.0875, 10.7381) -> (2.1484, 10.5594)
  line L738 (2.1484, 10.5594) -> (2.202, 10.3815)
  line L739 (2.202, 10.3815) -> (2.2482, 10.2044)
  line L740 (2.2482, 10.2044) -> (2.2867, 10.0284)
  line L741 (2.2867, 10.0284) -> (2.3172, 9.8537)
  line L742 (2.3172, 9.8537) -> (2.3391, 9.6806)
  line L743 (2.3391, 9.6806) -> (2.3516, 9.5094)
  line L744 (2.3516, 9.5094) -> (2.3535, 9.3406)
  line L745 (2.3535, 9.3406) -> (2.3417, 9.1751)
  line L746 (2.3417, 9.1751) -> (2.3121, 9.0141)
  line L747 (2.3121, 9.0141) -> (2.3008, 8.9327)
  line L748 (2.3008, 8.9327) -> (2.2948, 8.8499)
  line L749 (2.2948, 8.8499) -> (2.2952, 8.7654)
  line L750 (2.2952, 8.7654) -> (2.3043, 8.6786)
  line L751 (2.3043, 8.6786) -> (2.3133, 8.6339)
  line L752 (2.3133, 8.6339) -> (2.3267, 8.588)
  line L753 (2.3267, 8.588) -> (2.3467, 8.5402)
  line L754 (2.3467, 8.5402) -> (2.3785, 8.489)
  line L755 (2.3785, 8.489) -> (2.4779, 8.418)
  line L756 (2.4779, 8.418) -> (2.9433, 8.2667)
  line L757 (2.9433, 8.2667) -> (3.0655, 8.2658)
  line L758 (3.0655, 8.2658) -> (3.1213, 8.2885)
  line L759 (3.1213, 8.2885) -> (3.1655, 8.3154)
  line L760 (3.1655, 8.3154) -> (3.2033, 8.3447)
  line L761 (3.2033, 8.3447) -> (3.2369, 8.3755)
  line L762 (3.2369, 8.3755) -> (3.2953, 8.4404)
  line L763 (3.2953, 8.4404) -> (3.3453, 8.5086)
  line L764 (3.3453, 8.5086) -> (3.3891, 8.5791)
  line L765 (3.3891, 8.5791) -> (3.4279, 8.6515)
  line L766 (3.4279, 8.6515) -> (3.4985, 8.7992)
  line L767 (3.4985, 8.7992) -> (3.5863, 8.94)
  line L768 (3.5863, 8.94) -> (3.687, 9.0755)
  line L769 (3.687, 9.0755) -> (3.7977, 9.2066)
  line L770 (3.7977, 9.2066) -> (3.9172, 9.3338)
  line L771 (3.9172, 9.3338) -> (4.0445, 9.4573)
  line L772 (4.0445, 9.4573) -> (4.1792, 9.577)
  line L773 (4.1792, 9.577) -> (4.3207, 9.6931)
  line L774 (4.3207, 9.6931) -> (4.4686, 9.8055)
  line L775 (4.4686, 9.8055) -> (4.6228, 9.9143)
  line L776 (4.6228, 9.9143) -> (4.783, 10.0193)
  line L777 (4.783, 10.0193) -> (4.907, 10.0956)
  line L778 (4.907, 10.0956) -> (5.2832, 9.9038)
  line L779 (5.2832, 9.9038) -> (5.2944, 9.7587)
  line L780 (5.2944, 9.7587) -> (5.3036, 9.5674)
  line L781 (5.3036, 9.5674) -> (5.3063, 9.3788)
  line L782 (5.3063, 9.3788) -> (5.3023, 9.1929)
  line L783 (5.3023, 9.1929) -> (5.2915, 9.0102)
  line L784 (5.2915, 9.0102) -> (5.2737, 8.8309)
  line L785 (5.2737, 8.8309) -> (5.2487, 8.6554)
  line L786 (5.2487, 8.6554) -> (5.2161, 8.484)
  line L787 (5.2161, 8.484) -> (5.1751, 8.3173)
  line L788 (5.1751, 8.3173) -> (5.1247, 8.1562)
  line L789 (5.1247, 8.1562) -> (5.0624, 8.0024)
  line L790 (5.0624, 8.0024) -> (4.9844, 7.8585)
  line L791 (4.9844, 7.8585) -> (4.9486, 7.7845)
  line L792 (4.9486, 7.7845) -> (4.9172, 7.7076)
  line L793 (4.9172, 7.7076) -> (4.8915, 7.6271)
  line L794 (4.8915, 7.6271) -> (4.8733, 7.5417)
  line L795 (4.8733, 7.5417) -> (4.8681, 7.4964)
  line L796 (4.8681, 7.4964) -> (4.8667, 7.4486)
  line L797 (4.8667, 7.4486) -> (4.8709, 7.3971)
  line L798 (4.8709, 7.3971) -> (4.8853, 7.3385)
  line L799 (4.8853, 7.3385) -> (4.9579, 7.2403)
  line L800 (4.9579, 7.2403) -> (5.3538, 6.9526)
  line L801 (5.3538, 6.9526) -> (5.4697, 6.914)
  line L802 (5.4697, 6.914) -> (5.5298, 6.9183)
  line L803 (5.5298, 6.9183) -> (5.5802, 6.9303)
  line L804 (5.5802, 6.9303) -> (5.6252, 6.9464)
  line L805 (5.6252, 6.9464) -> (5.6667, 6.9653)
  line L806 (5.6667, 6.9653) -> (5.7423, 7.009)
  line L807 (5.7423, 7.009) -> (5.8109, 7.0584)
  line L808 (5.8109, 7.0584) -> (5.8743, 7.1119)
  line L809 (5.8743, 7.1119) -> (5.9336, 7.1688)
  line L810 (5.9336, 7.1688) -> (6.0464, 7.2875)
  line L811 (6.0464, 7.2875) -> (6.1734, 7.3943)
  line L812 (6.1734, 7.3943) -> (6.311, 7.492)
  line L813 (6.311, 7.492) -> (6.4569, 7.5825)
  line L814 (6.4569, 7.5825) -> (6.6098, 7.6665)
  line L815 (6.6098, 7.6665) -> (6.769, 7.7445)
  line L816 (6.769, 7.7445) -> (6.9341, 7.8168)
  line L817 (6.9341, 7.8168) -> (7.1045, 7.8835)
  line L818 (7.1045, 7.8835) -> (7.28, 7.9447)
  line L819 (7.28, 7.9447) -> (7.4603, 8.0005)
  line L820 (7.4603, 8.0005) -> (7.6451, 8.0509)
  line L821 (7.6451, 8.0509) -> (7.7865, 8.0851)
  line L822 (7.7865, 8.0851) -> (8.0851, 7.7865)
  line L823 (8.0851, 7.7865) -> (8.0509, 7.6451)
  line L824 (8.0509, 7.6451) -> (8.0005, 7.4603)
  line L825 (8.0005, 7.4603) -> (7.9447, 7.28)
  line L826 (7.9447, 7.28) -> (7.8835, 7.1045)
  line L827 (7.8835, 7.1045) -> (7.8168, 6.9341)
  line L828 (7.8168, 6.9341) -> (7.7445, 6.769)
  line L829 (7.7445, 6.769) -> (7.6665, 6.6098)
  line L830 (7.6665, 6.6098) -> (7.5825, 6.4569)
  line L831 (7.5825, 6.4569) -> (7.492, 6.311)
  line L832 (7.492, 6.311) -> (7.3943, 6.1734)
  line L833 (7.3943, 6.1734) -> (7.2875, 6.0464)
  line L834 (7.2875, 6.0464) -> (7.1688, 5.9336)
  line L835 (7.1688, 5.9336) -> (7.1119, 5.8743)
  line L836 (7.1119, 5.8743) -> (7.0584, 5.8109)
  line L837 (7.0584, 5.8109) -> (7.009, 5.7423)
  line L838 (7.009, 5.7423) -> (6.9653, 5.6667)
  line L839 (6.9653, 5.6667) -> (6.9464, 5.6252)
  line L840 (6.9464, 5.6252) -> (6.9303, 5.5802)
  line L841 (6.9303, 5.5802) -> (6.9183, 5.5298)
  line L842 (6.9183, 5.5298) -> (6.914, 5.4697)
  line L843 (6.914, 5.4697) -> (6.9526, 5.3538)
  line L844 (6.9526, 5.3538) -> (7.2403, 4.9579)
  line L845 (7.2403, 4.9579) -> (7.3385, 4.8853)
  line L846 (7.3385, 4.8853) -> (7.3971, 4.8709)
  line L847 (7.3971, 4.8709) -> (7.4486, 4.8667)
  line L848 (7.4486, 4.8667) -> (7.4964, 4.8681)
  line L849 (7.4964, 4.8681) -> (7.5417, 4.8733)
  line L850 (7.5417, 4.8733) -> (7.6271, 4.8915)
  line L851 (7.6271, 4.8915) -> (7.7076, 4.9172)
  line L852 (7.7076, 4.9172) -> (7.7845, 4.9486)
  line L853 (7.7845, 4.9486) -> (7.8585, 4.9844)
  line L854 (7.8585, 4.9844) -> (8.0024, 5.0624)
  line L855 (8.0024, 5.0624) -> (8.1562, 5.1247)
  line L856 (8.1562, 5.1247) -> (8.3173, 5.1751)
  line L857 (8.3173, 5.1751) -> (8.484, 5.2161)
  line L858 (8.484, 5.2161) -> (8.6554, 5.2487)
  line L859 (8.6554, 5.2487) -> (8.8309, 5.2738)
  line L860 (8.8309, 5.2738) -> (9.0102, 5.2915)
  line L861 (9.0102, 5.2915) -> (9.1929, 5.3023)
  line L862 (9.1929, 5.3023) -> (9.3788, 5.3063)
  line L863 (9.3788, 5.3063) -> (9.5674, 5.3036)
  line L864 (9.5674, 5.3036) -> (9.7587, 5.2944)
  line L865 (9.7587, 5.2944) -> (9.9038, 5.2832)
  line L866 (9.9038, 5.2832) -> (10.0956, 4.907)
  line L867 (10.0956, 4.907) -> (10.0193, 4.783)
  line L868 (10.0193, 4.783) -> (9.9143, 4.6228)
  line L869 (9.9143, 4.6228) -> (9.8055, 4.4686)
  line L870 (9.8055, 4.4686) -> (9.6931, 4.3207)
  line L871 (9.6931, 4.3207) -> (9.577, 4.1792)
  line L872 (9.577, 4.1792) -> (9.4573, 4.0445)
  line L873 (9.4573, 4.0445) -> (9.3338, 3.9172)
  line L874 (9.3338, 3.9172) -> (9.2066, 3.7977)
  line L875 (9.2066, 3.7977) -> (9.0755, 3.687)
  line L876 (9.0755, 3.687) -> (8.94, 3.5863)
  line L877 (8.94, 3.5863) -> (8.7992, 3.4985)
  line L878 (8.7992, 3.4985) -> (8.6516, 3.4279)
  line L879 (8.6516, 3.4279) -> (8.5791, 3.3891)
  line L880 (8.5791, 3.3891) -> (8.5086, 3.3453)
  line L881 (8.5086, 3.3453) -> (8.4404, 3.2953)
  line L882 (8.4404, 3.2953) -> (8.3755, 3.2369)
  line L883 (8.3755, 3.2369) -> (8.3447, 3.2033)
  line L884 (8.3447, 3.2033) -> (8.3154, 3.1655)
  line L885 (8.3154, 3.1655) -> (8.2885, 3.1213)
  line L886 (8.2885, 3.1213) -> (8.2658, 3.0655)
  line L887 (8.2658, 3.0655) -> (8.2667, 2.9433)
  line L888 (8.2667, 2.9433) -> (8.418, 2.4779)
  circle A2 centre (0, 0) radius 0.5
  line L889 (-7.9358, -7.9358) -> (7.9358, 7.9358) construction
  line L890 (7.9358, -7.9358) -> (-7.9358, 7.9358) construction
  dimension "d7" = 1
  dimension "d6" = 1
  dimension "d8" = 1
  constraints: 16 end point, 4 collinear, 2 coincident, 2 parallel, 1 midpoint, 25 other
  measures "d6" distance between parallel lines of L1 L2
  measures "d8" distance between parallel lines of L6 L5